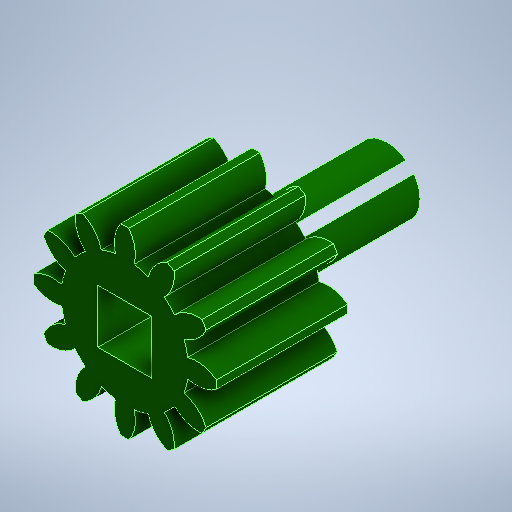
# Autodesk Inventor part: Pinion Gear
Saved by Autodesk Inventor 2025.4 (Build 294407000, 407)
## iProperties
Created: 2026-04-04
Part Number: Pinion Gear
Material: Generic
Document SubType Name: Modeling
Designer: lenovo
Density: 1 g/cm^3
Appearance: Default(1)
Author: lenovo
Autodesk Inventor part; units mm, degrees
ref_plane "YZ Plane" through (0, 0, 0) normal (1, 0, 0) x (0, 1, 0)
ref_plane "XZ Plane" through (0, 0, 0) normal (0, 1, 0) x (-1, 0, 0)
ref_plane "XY Plane" through (0, 0, 0) normal (0, 0, 1) x (1, 0, 0)
sketch "Sketch1" plane through (0, 0, 0) normal (0, 0, 1) x (1, 0, 0)
  circle A0 centre (0, 0) radius 2.5
  dimension "d0" = 5
  constraints: 1 centre point, 1 coincident
  measures "d0" diameter of A0
extrude "Extrusion1" add sketch "Sketch1" along normal blind 10
sketch "Sketch2" plane through (0, 0, 10) normal (0, 0, 1) x (1, 0, 0)
  circle A0 centre (0, 0) radius 6.99
  circle A1 centre (0, 0) radius 4.85
  line L0 (-6.99, 0) -> (6.99, 0)
  arc A2 (6.9831, 0.31) -> (4.7977, 0.71) centre (5.4872, -1.6931) ccw
  arc A3 (4.7977, -0.71) -> (6.9831, -0.31) centre (5.4872, 1.6931) ccw
  point P0 (4.8336, 0.3987)
  point P1 (4.7977, -0.71)
  point P2 (6.9831, -0.31)
  dimension "d3" = 13.98
  dimension "d17" = 9.7
  dimension "d18" = 0.62
  dimension "d19" = 1.42
  dimension "d20" = 2.5
  constraints: 9 point on circle, 4 centre point, 3 coincident, 3 symmetric about line, 2 end point, 1 horizontal, 1 midpoint, 1 other
  measures "d3" diameter of A0
  measures "d17" diameter of A1
  measures "d18" distance of A3.end A2.start
  measures "d19" distance of A1.end A3.start
  measures "d20" radius of A2
extrude "Extrusion2" add sketch "Sketch2" along normal blind 10 contours L0 A1 | A1 L0
extrude "Extrusion3" add sketch "Sketch2" along normal up to surface (10 mm away) contours L0 A1 A2 A0 | A0 A3 A1 L0 | L0 A1 | A1 L0 picked at (6.1088, 0.1995) picked at (6.1089, -0.1995)
pattern_circular "Circular Pattern1" count 12 over 360 about axis through (0, 0, -10) along (0, 0, 1) of "Extrusion3"
sketch "Sketch3" plane through (0, 0, 20) normal (0, 0, 1) x (1, 0, 0)
  line L0 (-2.04, -2.04) -> (2.04, -2.04)
  line L1 (2.04, -2.04) -> (2.04, 2.04)
  line L2 (2.04, 2.04) -> (-2.04, 2.04)
  line L3 (-2.04, 2.04) -> (-2.04, -2.04)
  line L4 (-2.04, -2.04) -> (2.04, 2.04) construction
  line L5 (2.04, -2.04) -> (-2.04, 2.04) construction
  point P0 (0, 0)
  dimension "d22" = 4.08
  constraints: 12 end point, 2 midpoint, 2 parallel, 2 perpendicular, 1 horizontal
  measures "d22" distance of L2.end L1.end
extrude "Extrusion4" cut sketch "Sketch3" against normal through all
body "Solid1"
